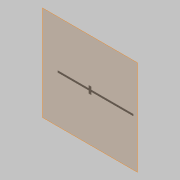
# Autodesk Inventor part: Dead reckoning line
Saved by Autodesk Inventor 2015 (Build 190159000, 159)
## iProperties
Created: 2015-08-13
Part Number: Dead reckoning line
Material: Generic
Document SubType Name: Modeling
Designer: v2jovano
Density: 1 g/cm^3
Appearance: Default
Author: v2jovano
Autodesk Inventor part; units mm, degrees
ref_plane "YZ Plane" through (0, 0, 0) normal (1, 0, 0) x (0, 1, 0)
ref_plane "XZ Plane" through (0, 0, 0) normal (0, 1, 0) x (-1, 0, 0)
ref_plane "XY Plane" through (0, 0, 0) normal (0, 0, 1) x (1, 0, 0)
ref_plane "Work Plane1" through (0, 0, 0) normal (0, 0, 1) x (1, 0, 0)
sketch "Sketch1" plane through (0, 0, 0) normal (0, 0, 1) x (1, 0, 0)
  line L0 (1219.2, 1219.2) -> (-1219.2, 1219.2) projected
  line L1 (-1219.2, 1231.9) -> (-1219.2, -1231.9) projected
  line L2 (1219.2, -1231.9) -> (1219.2, 1231.9) projected
  line L3 (-1219.2, -1219.2) -> (1219.2, -1219.2) projected
  line L4 (-914.4, -406.4) -> (-914.4, 406.4) projected
  line L5 (-914.4, 25.4) -> (1219.2, 25.4)
  line L6 (1219.2, 25.4) -> (1219.2, -25.4)
  line L7 (1219.2, -25.4) -> (-914.4, -25.4)
  line L8 (-914.4, -25.4) -> (-914.4, 25.4)
  line L9 (-38.1, 101.6) -> (38.1, 101.6)
  line L10 (38.1, 101.6) -> (38.1, -101.6)
  line L11 (38.1, -101.6) -> (-38.1, -101.6)
  line L12 (-38.1, -101.6) -> (-38.1, 101.6)
  point P0 (0, 0)
  dimension "d0" = 50.8
  dimension "d1" = 25.4
  dimension "d2" = 76.2
  dimension "d3" = 38.1
  dimension "d4" = 203.2
  dimension "d5" = 101.6
  constraints: 16 end point, 4 parallel, 2 horizontal, 2 perpendicular, 2 point on line
  measures "d0" distance between parallel lines of L7 L5
  measures "d1" distance from line of L5 point (0, 0)
  measures "d2" distance between parallel lines of L10 L12
  measures "d3" distance from line of point (0, 0) L10
  measures "d4" distance between parallel lines of L11 L9
  measures "d5" distance from line of L9 point (0, 0)
extrude "Extrusion1" add sketch "Sketch1" against normal blind 6.35 contours L2 L7 L10 L5 | L10 L7 L12 L5 | L5 L12 L9 L10 | L10 L11 L12 L7 | L12 L7 L4 L5
equation "\"d1\" = 0.5 * d0"
equation "\"d5\" = 0.5 * d4"
body "Solid1"
